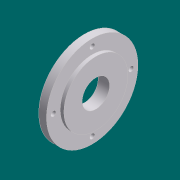
# Autodesk Inventor part: P04
Saved by Autodesk Inventor 2012 SP1 (Build 160190100, 190)
## iProperties
Created: 2011-05-11
Material: Aluminium
Document SubType Name: Modeling
Designer: sta
Density: 2.7 g/cm^3
Description: Deckel M0,7
Mass: 20.1757 g
Surface Area: 36.4525 cm^2
Volume: 7.47247 cm^3
Part Number: P04
Title: Kart
Author: sta
Autodesk Inventor part; units mm, degrees
ref_plane "YZ Plane" through (0, 0, 0) normal (1, 0, 0) x (0, 1, 0)
ref_plane "XZ Plane" through (0, 0, 0) normal (0, 1, 0) x (-1, 0, 0)
ref_plane "XY Plane" through (0, 0, 0) normal (0, 0, 1) x (1, 0, 0)
sketch "Sketch1" plane through (0, 0, 0) normal (0, 0, 1) x (1, 0, 0)
  line L0 (-11.0022, 0) -> (11.0022, 0) construction
  line L1 (0, 10.3849) -> (0, -10.3849) construction
  line L2 (0, 0) -> (0, 20)
  line L3 (0, 20) -> (3.4, 20)
  line L4 (3.4, 20) -> (3.4, 14)
  line L5 (3.4, 14) -> (5, 14)
  line L6 (5, 14) -> (5, 0)
  line L7 (5, 0) -> (0, 0)
  line L8 (0, 6) -> (5, 6)
  dimension "d0" = 40
  dimension "d1" = 28
  dimension "d2" = 1.6
  dimension "d4" = 12
  dimension "d17" = 5
  constraints: 18 end point, 3 parallel, 3 perpendicular, 3 point on line, 2 collinear, 2 midpoint, 1 coincident, 1 horizontal
  measures "d0" diameter of L3 L0
  measures "d1" diameter of L5 L0
  measures "d2" distance between parallel lines of L4 L6
  measures "d4" diameter of L8 L0
  measures "d17" distance between parallel lines of L6 L2
revolve "Revolution1" add sketch "Sketch1" angle 360 about axis through (-11.0022, 0, 0) along (1, 0, 0) contours L2 L3 L4 L5 L6 L8
sketch "Sketch2" plane through (0, 0, 0) normal (-1, 0, 0) x (0, 0, 1)
  circle A0 centre (0, 0) radius 17 construction
  line L0 (0, 0) -> (-21.4597, 0) construction
  point P0 (-17, 0)
  dimension "d6" = 34
  constraints: 2 end point, 1 coincident, 1 horizontal, 1 horizontal alignment, 1 point on line, 2 other
hole "Hole1" at (0, 0, -17) direction (1, 0, 0) diameter 2.2 depth 8 tip angle 118
pattern_circular "Circular Pattern1" count 4 over 360 about axis through (2.5, 0, 0) along (1, 0, 0) of "Hole1"
body "Solid1"
